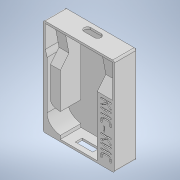
# Autodesk Inventor part: Корпус
Saved by Autodesk Inventor 2021.2 (Build 252289000, 289)
## iProperties
Created: 2023-10-18
Part Number: Корпус
Material: Типовые
Document SubType Name: Modeling
Designer: DELL
Density: 1 g/cm^3
Appearance: По умолчанию
Author: DELL
Autodesk Inventor part; units mm, degrees
ref_plane "YZ Plane" through (0, 0, 0) normal (1, 0, 0) x (0, 1, 0)
ref_plane "XZ Plane" through (0, 0, 0) normal (0, 1, 0) x (-1, 0, 0)
ref_plane "XY Plane" through (0, 0, 0) normal (0, 0, 1) x (1, 0, 0)
sketch "Эскиз1" plane through (0, 0, 0) normal (0, 0, 1) x (1, 0, 0)
  line L0 (10.25, -26.5) -> (-10.25, -26.5) construction
  line L1 (-10.25, -26.5) -> (-10.25, 26.5) construction
  line L2 (-10.25, 26.5) -> (10.25, 26.5) construction
  line L3 (10.25, 26.5) -> (10.25, -26.5) construction
  line L4 (10.25, -26.5) -> (-10.25, 26.5) construction
  line L5 (-10.25, -26.5) -> (10.25, 26.5) construction
  line L6 (19, 14.5) -> (-19, 14.5) construction
  line L7 (-19, 14.5) -> (-19, 26.5) construction
  line L8 (-19, 26.5) -> (19, 26.5) construction
  line L9 (19, 26.5) -> (19, 14.5) construction
  line L10 (19, 14.5) -> (-19, 26.5) construction
  line L11 (-19, 14.5) -> (19, 26.5) construction
  line L12 (-19.5, 14) -> (-10.75, 14)
  line L13 (-10.75, 14) -> (-10.75, -27)
  line L14 (-10.75, -27) -> (10.75, -27)
  line L15 (10.75, -27) -> (10.75, 14)
  line L16 (10.75, 14) -> (19.5, 14)
  line L17 (19.5, 14) -> (19.5, 27)
  line L18 (19.5, 27) -> (-19.5, 27)
  line L19 (-19.5, 27) -> (-19.5, 14)
  line L20 (0, 26.5) -> (0, -26.5) construction
  line L21 (20.7, -28.2) -> (-20.7, -28.2)
  line L22 (-20.7, -28.2) -> (-20.7, 28.2)
  line L23 (-20.7, 28.2) -> (20.7, 28.2)
  line L24 (20.7, 28.2) -> (20.7, -28.2)
  line L25 (20.7, -28.2) -> (-20.7, 28.2) construction
  line L26 (-20.7, -28.2) -> (20.7, 28.2) construction
  line L27 (-10.75, 14) -> (-10.75, 27)
  line L28 (10.75, 14) -> (10.75, 27)
  point P0 (0, 0)
  point P1 (0, 20.5)
  point P2 (0, 20.5)
  point P3 (0, 0)
  point P4 (0, 0)
  dimension "d0" = 20.5
  dimension "d1" = 53
  dimension "d2" = 38
  dimension "d3" = 12
  dimension "d4" = 0
  dimension "d5" = 0.5
  dimension "d8" = 0.5
  dimension "d9" = 0.5
  dimension "d10" = 0.5
  dimension "d11" = 0.5
  dimension "d13" = 1.2
  dimension "d14" = 1.2
  dimension "d15" = 1.2
  constraints: 60 end point, 11 midpoint, 10 perpendicular, 7 parallel, 5 horizontal, 3 point on line, 1 vertical alignment, 2 other
  measures "d0" distance of L1.end L2.end
  measures "d1" distance of L0.end L1.end
  measures "d2" distance of L7.end L8.end
  measures "d3" distance of L6.end L7.end
  measures "d4" distance between parallel lines of L2 L8
  measures "d5" distance between parallel lines of L19 L7
  measures "d8" distance between parallel lines of L18 L8
  measures "d9" distance between parallel lines of L6 L12
  measures "d10" distance between parallel lines of L1 L13
  measures "d11" distance between parallel lines of L0 L14
  measures "d13" distance between parallel lines of L23 L18
  measures "d14" distance between parallel lines of L22 L19
  measures "d15" distance between parallel lines of L14 L21
extrude "Выдавливание1" add sketch "Эскиз1" along normal blind 7 contours L19 L18 L27 L12 | L18 L17 L16 L28 | L21 L22 L23 L24
extrude "Выдавливание2" add sketch "Эскиз1" along normal blind 5 from surface at 7
extrude "Выдавливание3" add sketch "Эскиз1" against normal blind 1 contours L19 L18 L27 L12 | L27 L18 L28 L15 L14 L13 | L18 L17 L16 L28 | L21 L22 L23 L24
fillet "Сопряжение1" radius 1 4 edges at (-20.7, 28.2, 5.5) (20.7, 28.2, 5.5) (-20.7, -28.2, 5.5) (20.7, -28.2, 5.5)
chamfer "Фаска1" distance 0.5 angle 45 8 edges at (20.7, 0, -1) (20.4071, -27.9071, -1) (0, -28.2, -1) (-20.4071, -27.9071, -1) (-20.7, 0, -1) (-20.4071, 27.9071, -1) (0, 28.2, -1) (20.4071, 27.9071, -1)
sketch "Эскиз2" plane through (-19.7, 28.2, 12) normal (0, 1, 0) x (1, 0, 0)
  line L0 (8.95, 12) -> (30.45, 12) construction
  line L1 (8.95, 12) -> (8.95, 5) construction
  line L2 (30.45, 12) -> (30.45, 5) construction
  line L3 (22.7, 8) -> (16.7, 8) construction
  line L4 (22.7, 10) -> (16.7, 10)
  line L5 (16.7, 6) -> (22.7, 6)
  arc A0 (22.7, 6) -> (22.7, 10) centre (22.7, 8) ccw
  arc A1 (16.7, 10) -> (16.7, 6) centre (16.7, 8) ccw
  point P0 (19.7, 12)
  point P1 (19.7, 8)
  point P2 (19.7, 12)
  dimension "d26" = 10
  dimension "d27" = 4
  dimension "d28" = 2
  constraints: 8 end point, 4 point on circle, 4 tangent, 2 centre point, 2 midpoint, 2 parallel, 1 vertical alignment
  measures "d27" distance between parallel lines of L5 L4
  measures "d28" distance between parallel lines of L4 L0
extrude "Выдавливание4" cut sketch "Эскиз2" against normal up to next
sketch "Эскиз3" plane through (-19.7, 28.2, 12) normal (0, 0, 1) x (1, 0, 0)
  line L0 (38.5472, -21.4883) -> (38.5472, -54.373) construction
  line L1 (38.5472, -54.373) -> (33.4021, -54.373) construction
  line L2 (33.4021, -54.373) -> (33.4021, -21.4883) construction
  line L3 (33.4021, -21.4883) -> (38.5472, -21.4883) construction
  line L4 (39.4, -56.4) -> (0, -56.4) construction
  line L5 (19.7, -56.4) -> (19.7, 0) construction
  line L6 (16.7, 0) -> (22.7, 0) construction
  line L7 (35.5501, -23.5132) -> (34.7542, -22.8483)
  line L8 (34.7542, -22.8483) -> (32.83, -22.8483)
  spline S0 degree 2 poles (32.83, -22.8483) (32.4472, -22.8483) (32.4472, -22.4655) knots 0 0 0 1 1 1
  spline S1 degree 2 poles (32.4472, -22.4655) (32.4472, -22.0827) (32.83, -22.0827) knots 0 0 0 1 1 1
  line L9 (32.83, -22.0827) -> (38.1694, -22.0827)
  spline S2 degree 2 poles (38.1694, -22.0827) (38.5472, -22.0827) (38.5472, -22.4655) knots 0 0 0 1 1 1
  spline S3 degree 2 poles (38.5472, -22.4655) (38.5472, -22.8483) (38.1694, -22.8483) knots 0 0 0 1 1 1
  line L10 (38.1694, -22.8483) -> (35.7616, -22.8483)
  line L11 (35.7616, -22.8483) -> (38.4213, -25.1453)
  spline S4 degree 2 poles (38.4213, -25.1453) (38.5472, -25.2561) (38.5472, -25.4324) knots 0 0 0 1 1 1
  spline S5 degree 2 poles (38.5472, -25.4324) (38.5472, -25.8152) (38.1694, -25.8152) knots 0 0 0 1 1 1
  spline S6 degree 2 poles (38.1694, -25.8152) (38.0233, -25.8152) (37.8823, -25.5886) knots 0 0 0 1 1 1
  line L12 (37.8823, -25.5886) -> (36.089, -24.0371)
  line L13 (36.089, -24.0371) -> (33.0164, -25.7598)
  spline S7 degree 2 poles (33.0164, -25.7598) (32.9257, -25.8152) (32.83, -25.8152) knots 0 0 0 1 1 1
  spline S8 degree 2 poles (32.83, -25.8152) (32.6789, -25.8152) (32.4472, -25.5785) (32.4472, -25.4324) knots 0 0 0 1 2 2 2
  spline S9 degree 2 poles (32.4472, -25.4324) (32.4472, -25.2007) (32.694, -25.0798) knots 0 0 0 1 1 1
  line L14 (32.694, -25.0798) -> (35.5501, -23.5132)
  spline S10 degree 2 poles (38.5472, -30.1774) (38.5472, -30.5602) (38.1694, -30.5602) knots 0 0 0 1 1 1
  line L15 (38.1694, -30.5602) -> (32.83, -30.5602)
  spline S11 degree 2 poles (32.83, -30.5602) (32.4472, -30.5602) (32.4472, -30.1774) knots 0 0 0 1 1 1
  spline S12 degree 2 poles (32.4472, -30.1774) (32.4472, -29.7946) (32.83, -29.7946) knots 0 0 0 1 1 1
  line L16 (32.83, -29.7946) -> (36.6985, -29.7946)
  line L17 (36.6985, -29.7946) -> (33.102, -27.5984)
  spline S13 degree 2 poles (33.102, -27.5984) (32.7998, -27.5984) (32.699, -27.5682) knots 0 0 0 1 1 1
  spline S14 degree 2 poles (32.699, -27.5682) (32.4472, -27.5027) (32.4472, -27.2156) knots 0 0 0 1 1 1
  spline S15 degree 2 poles (32.4472, -27.2156) (32.4472, -26.8327) (32.83, -26.8327) knots 0 0 0 1 1 1
  line L18 (32.83, -26.8327) -> (38.1694, -26.8327)
  spline S16 degree 2 poles (38.1694, -26.8327) (38.5472, -26.8327) (38.5472, -27.2156) knots 0 0 0 1 1 1
  spline S17 degree 2 poles (38.5472, -27.2156) (38.5472, -27.5984) (38.1694, -27.5984) knots 0 0 0 1 1 1
  line L19 (38.1694, -27.5984) -> (34.3009, -27.5984)
  line L20 (34.3009, -27.5984) -> (37.8974, -29.7946)
  spline S18 degree 2 poles (37.8974, -29.7946) (38.1996, -29.7946) (38.2953, -29.8198) knots 0 0 0 1 1 1
  spline S19 degree 2 poles (38.2953, -29.8198) (38.5472, -29.8853) (38.5472, -30.1774) knots 0 0 0 1 1 1
  spline S20 degree 2 poles (38.5472, -34.3381) (38.5472, -34.7209) (38.1694, -34.7209) knots 0 0 0 1 1 1
  spline S21 degree 2 poles (38.1694, -34.7209) (37.7866, -34.7209) (37.7866, -34.3381) knots 0 0 0 1 1 1
  line L21 (37.7866, -34.3381) -> (37.7866, -33.1544)
  spline S22 degree 2 poles (37.7866, -33.1544) (37.7866, -32.6909) (37.3886, -32.4592) knots 0 0 0 1 1 1
  spline S23 degree 2 poles (37.3886, -32.4592) (37.2023, -32.3484) (36.9806, -32.3484) knots 0 0 0 1 1 1
  line L22 (36.9806, -32.3484) -> (34.0188, -32.3484)
  spline S24 degree 2 poles (34.0188, -32.3484) (33.6813, -32.3484) (33.2078, -32.8219) (33.2078, -33.1544) knots 0 0 0 1 2 2 2
  line L23 (33.2078, -33.1544) -> (33.2078, -34.3381)
  spline S25 degree 2 poles (33.2078, -34.3381) (33.2078, -34.7209) (32.83, -34.7209) knots 0 0 0 1 1 1
  spline S26 degree 2 poles (32.83, -34.7209) (32.4472, -34.7209) (32.4472, -34.3381) knots 0 0 0 1 1 1
  line L24 (32.4472, -34.3381) -> (32.4472, -33.1544)
  spline S27 degree 2 poles (32.4472, -33.1544) (32.4472, -32.4995) (33.3639, -31.5828) (34.0188, -31.5828) knots 0 0 0 1 2 2 2
  line L25 (34.0188, -31.5828) -> (36.9857, -31.5828)
  spline S28 degree 2 poles (36.9857, -31.5828) (37.6304, -31.5828) (38.5472, -32.4995) (38.5472, -33.1544) knots 0 0 0 1 2 2 2
  line L26 (38.5472, -33.1544) -> (38.5472, -34.3381)
  line L27 (33.9281, -38.4938) -> (33.9281, -36.1213)
  spline S29 degree 2 poles (33.9281, -36.1213) (33.9281, -35.7384) (34.3109, -35.7384) knots 0 0 0 1 1 1
  spline S30 degree 2 poles (34.3109, -35.7384) (34.6887, -35.7384) (34.6887, -36.1213) knots 0 0 0 1 1 1
  line L28 (34.6887, -36.1213) -> (34.6887, -38.4938)
  spline S31 degree 2 poles (34.6887, -38.4938) (34.6887, -38.8766) (34.3109, -38.8766) knots 0 0 0 1 1 1
  spline S32 degree 2 poles (34.3109, -38.8766) (33.9281, -38.8766) (33.9281, -38.4938) knots 0 0 0 1 1 1
  line L29 (35.5501, -41.3246) -> (34.7542, -40.6597)
  line L30 (34.7542, -40.6597) -> (32.83, -40.6597)
  spline S33 degree 2 poles (32.83, -40.6597) (32.4472, -40.6597) (32.4472, -40.2769) knots 0 0 0 1 1 1
  spline S34 degree 2 poles (32.4472, -40.2769) (32.4472, -39.8941) (32.83, -39.8941) knots 0 0 0 1 1 1
  line L31 (32.83, -39.8941) -> (38.1694, -39.8941)
  spline S35 degree 2 poles (38.1694, -39.8941) (38.5472, -39.8941) (38.5472, -40.2769) knots 0 0 0 1 1 1
  spline S36 degree 2 poles (38.5472, -40.2769) (38.5472, -40.6597) (38.1694, -40.6597) knots 0 0 0 1 1 1
  line L32 (38.1694, -40.6597) -> (35.7616, -40.6597)
  line L33 (35.7616, -40.6597) -> (38.4213, -42.9567)
  spline S37 degree 2 poles (38.4213, -42.9567) (38.5472, -43.0675) (38.5472, -43.2438) knots 0 0 0 1 1 1
  spline S38 degree 2 poles (38.5472, -43.2438) (38.5472, -43.6266) (38.1694, -43.6266) knots 0 0 0 1 1 1
  spline S39 degree 2 poles (38.1694, -43.6266) (38.0233, -43.6266) (37.8823, -43.4) knots 0 0 0 1 1 1
  line L34 (37.8823, -43.4) -> (36.089, -41.8485)
  line L35 (36.089, -41.8485) -> (33.0164, -43.5712)
  spline S40 degree 2 poles (33.0164, -43.5712) (32.9257, -43.6266) (32.83, -43.6266) knots 0 0 0 1 1 1
  spline S41 degree 2 poles (32.83, -43.6266) (32.6789, -43.6266) (32.4472, -43.3899) (32.4472, -43.2438) knots 0 0 0 1 2 2 2
  spline S42 degree 2 poles (32.4472, -43.2438) (32.4472, -43.0121) (32.694, -42.8912) knots 0 0 0 1 1 1
  line L36 (32.694, -42.8912) -> (35.5501, -41.3246)
  spline S43 degree 2 poles (38.5472, -47.9888) (38.5472, -48.3716) (38.1694, -48.3716) knots 0 0 0 1 1 1
  line L37 (38.1694, -48.3716) -> (32.83, -48.3716)
  spline S44 degree 2 poles (32.83, -48.3716) (32.4472, -48.3716) (32.4472, -47.9888) knots 0 0 0 1 1 1
  spline S45 degree 2 poles (32.4472, -47.9888) (32.4472, -47.606) (32.83, -47.606) knots 0 0 0 1 1 1
  line L38 (32.83, -47.606) -> (36.6985, -47.606)
  line L39 (36.6985, -47.606) -> (33.102, -45.4098)
  spline S46 degree 2 poles (33.102, -45.4098) (32.7998, -45.4098) (32.699, -45.3796) knots 0 0 0 1 1 1
  spline S47 degree 2 poles (32.699, -45.3796) (32.4472, -45.3141) (32.4472, -45.027) knots 0 0 0 1 1 1
  spline S48 degree 2 poles (32.4472, -45.027) (32.4472, -44.6441) (32.83, -44.6441) knots 0 0 0 1 1 1
  line L40 (32.83, -44.6441) -> (38.1694, -44.6441)
  spline S49 degree 2 poles (38.1694, -44.6441) (38.5472, -44.6441) (38.5472, -45.027) knots 0 0 0 1 1 1
  spline S50 degree 2 poles (38.5472, -45.027) (38.5472, -45.4098) (38.1694, -45.4098) knots 0 0 0 1 1 1
  line L41 (38.1694, -45.4098) -> (34.3009, -45.4098)
  line L42 (34.3009, -45.4098) -> (37.8974, -47.606)
  spline S51 degree 2 poles (37.8974, -47.606) (38.1996, -47.606) (38.2953, -47.6312) knots 0 0 0 1 1 1
  spline S52 degree 2 poles (38.2953, -47.6312) (38.5472, -47.6966) (38.5472, -47.9888) knots 0 0 0 1 1 1
  spline S53 degree 2 poles (38.5472, -52.1495) (38.5472, -52.5323) (38.1694, -52.5323) knots 0 0 0 1 1 1
  spline S54 degree 2 poles (38.1694, -52.5323) (37.7866, -52.5323) (37.7866, -52.1495) knots 0 0 0 1 1 1
  line L43 (37.7866, -52.1495) -> (37.7866, -50.9658)
  spline S55 degree 2 poles (37.7866, -50.9658) (37.7866, -50.5023) (37.3886, -50.2706) knots 0 0 0 1 1 1
  spline S56 degree 2 poles (37.3886, -50.2706) (37.2023, -50.1598) (36.9806, -50.1598) knots 0 0 0 1 1 1
  line L44 (36.9806, -50.1598) -> (34.0188, -50.1598)
  spline S57 degree 2 poles (34.0188, -50.1598) (33.6813, -50.1598) (33.2078, -50.6333) (33.2078, -50.9658) knots 0 0 0 1 2 2 2
  line L45 (33.2078, -50.9658) -> (33.2078, -52.1495)
  spline S58 degree 2 poles (33.2078, -52.1495) (33.2078, -52.5323) (32.83, -52.5323) knots 0 0 0 1 1 1
  spline S59 degree 2 poles (32.83, -52.5323) (32.4472, -52.5323) (32.4472, -52.1495) knots 0 0 0 1 1 1
  line L46 (32.4472, -52.1495) -> (32.4472, -50.9658)
  spline S60 degree 2 poles (32.4472, -50.9658) (32.4472, -50.3109) (33.3639, -49.3942) (34.0188, -49.3942) knots 0 0 0 1 2 2 2
  line L47 (34.0188, -49.3942) -> (36.9857, -49.3942)
  spline S61 degree 2 poles (36.9857, -49.3942) (37.6304, -49.3942) (38.5472, -50.3109) (38.5472, -50.9658) knots 0 0 0 1 2 2 2
  line L48 (38.5472, -50.9658) -> (38.5472, -52.1495)
  point P0 (19.7, -28.2)
  constraints: 2 end point, 2 midpoint, 2 other
emboss "Рельеф1" sketch "Эскиз3" operation cut depth 0.6 direction (0, 0, -1)
sketch "Эскиз4" plane through (-19.7, 28.2, 12) normal (0, 0, 1) x (1, 0, 0)
  line L0 (8.95, -14.2) -> (8.95, -55.2) construction
  line L1 (0.2, -1.2) -> (0.2, -14.2) construction
  line L2 (0.2, -1.2) -> (3.2, -1.2)
  line L3 (8.95, -1.2) -> (0.2, -1.2) construction
  line L4 (3.2, -1.2) -> (3.2, -14.2)
  line L5 (0.2, -14.2) -> (8.95, -14.2) construction
  line L6 (0.2, -14.2) -> (3.2, -14.2) construction
  line L7 (0.2, -14.2) -> (0.2, -1.2)
  line L8 (8.95, -55.2) -> (30.45, -55.2) construction
  line L9 (1.2, -17.8192) -> (1.2, -45.7113)
  line L10 (3.2, -37.8219) -> (3.2, -14.2)
  line L11 (1.2, -17.8192) -> (1.2, -16.0429) construction
  line L12 (1.2, -16.0429) -> (0.2, -15.3575) construction
  line L13 (0.2, -15.3575) -> (0.2, -14.2) construction
  spline S0 degree 3 poles (1.2, -17.8192) (1.2, -16.0429) (0.2, -15.3575) (0.2, -14.2) knots 1 1 1 1 2 2 2 2
  line L14 (8.95, -53.2) -> (3.0919, -52.2989) construction
  line L15 (3.0919, -52.2989) -> (1.2, -48.7736) construction
  line L16 (1.2, -48.7736) -> (1.2, -45.7113) construction
  spline S1 degree 3 poles (8.95, -53.2) (3.0919, -52.2989) (1.2, -48.7736) (1.2, -45.7113) knots 1 1 1 1 2 2 2 2
  line L17 (8.95, -41.2) -> (4.9393, -41.2) construction
  line L18 (4.9393, -41.2) -> (3.2, -39.7886) construction
  line L19 (3.2, -39.7886) -> (3.2, -37.8219) construction
  spline S2 degree 3 poles (8.95, -41.2) (4.9393, -41.2) (3.2, -39.7886) (3.2, -37.8219) knots 1 1 1 1 2 2 2 2
  line L20 (8.95, -53.2) -> (8.95, -41.2)
  point P0 (19.7, -28.2)
  point P1 (8.95, -18.2)
  point P2 (4.95, -14.2)
  dimension "d34" = 3
  dimension "d37" = 2
  dimension "d38" = 12
  dimension "d39" = 2
  constraints: 14 end point, 5 point on line, 5 vertical, 3 perpendicular, 1 collinear, 1 horizontal, 9 other
  measures "d34" distance of L1.start L2.end
  measures "d37" distance from line of L14.start L8
  measures "d38" distance of L17.start L14.start
  measures "d39" distance between parallel lines of L9 L10
extrude "Выдавливание5" cut sketch "Эскиз4" against normal up to surface (12 mm away)
sketch "Эскиз5" plane through (0, 0, 0) normal (1, 0, 0) x (0, 1, 0)
  line L0 (14, 12) -> (27, 12) construction
  line L1 (27, 12) -> (27, 7) construction
  line L2 (14, 7) -> (27, 7) construction
  line L3 (14, 7) -> (14, 12) construction
  line L4 (27, 9.5) -> (14, 7)
  line L5 (27, 7) -> (14, 7) construction
  line L6 (14, 7) -> (7.8507, 12)
  line L7 (7.8507, 12) -> (14, 12)
  line L8 (27.2, 12) -> (-27.2, 12) construction
  line L9 (14, 7) -> (14, 12)
  line L10 (27, 12) -> (27, 7) construction
  line L11 (27, 9.5) -> (27, 7)
  line L12 (27, 7) -> (14, 7)
  point P0 (0, 0)
  dimension "d42" = 130
  dimension "d43" = 2.5
  constraints: 12 end point, 2 midpoint, 2 point on line, 1 collinear, 1 perpendicular
  measures "d42" angle of L6 L4
  measures "d43" distance from line of L4.start L0
extrude "Выдавливание6" add sketch "Эскиз5" against normal up to surface (8.75 mm away) from surface at 19.5 contours L11 L12 L4
extrude "Выдавливание7" add sketch "Эскиз5" against normal up to surface (5.75 mm away) from surface at -10.75 contours L11 L12 L4
extrude "Выдавливание8" cut sketch "Эскиз5" along normal up to surface (19.5 mm away) contours L6 L7 L9
extrude "Выдавливание9" cut sketch "Эскиз5" against normal up to surface (16.5 mm away) contours L6 L7 L9
sketch "Эскиз6" plane through (-19.7, -28.2, 12) normal (0, -1, 0) x (1, 0, 0)
  line L0 (8.95, -12) -> (30.45, -12) construction
  line L1 (3.2, -12) -> (8.95, -12) construction
  line L2 (0.2, -12) -> (3.2, -12) construction
  line L3 (1.2, -12) -> (0.2, -12) construction
  line L4 (8.95, -12) -> (1.2, -12) construction
  line L5 (30.45, -12) -> (8.95, -12) construction
  line L6 (14.62, -3) -> (24.78, -3)
  line L7 (24.78, -3) -> (24.78, -7)
  line L8 (24.78, -7) -> (14.62, -7)
  line L9 (14.62, -7) -> (14.62, -3)
  point P0 (19.7, -12)
  point P1 (19.7, -12)
  point P2 (19.7, -7)
  dimension "d52" = 10.16
  dimension "d53" = 5
  dimension "d54" = 4
  constraints: 8 end point, 2 midpoint, 2 parallel, 1 horizontal, 1 perpendicular, 1 vertical alignment
  measures "d52" distance of L7.end L8.end
  measures "d53" distance between parallel lines of L0 L8
  measures "d54" distance of L8.end L6.start
extrude "Выдавливание10" cut sketch "Эскиз6" against normal up to next
equation "\"d8\" = d5"
equation "\"d9\" = d5"
equation "\"d10\" = d5"
equation "\"d11\" = d5"
equation "\"d14\" = d13"
equation "\"d15\" = d13"
